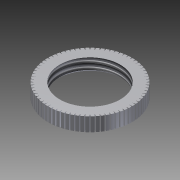
# Autodesk Inventor part: AT504M
Saved by Autodesk Inventor 2011 SP1 (Build 150282100, 282)
## iProperties
Created: 2013-12-24
Part Number: AT504M
Catalog Web Link: www.cadenas.de
Description: AT504M-Knurled Face Nut
Vendor: NKKSWITCHES
Document SubType Name: Modeling
Designer: PARTuser1
Manufacturer: NKKSWITCHES
Density: 1 g/cm^3
Category: PARTsolutions
Company: NKKSWITCHES
Title: AT504M
Author: Cadenas PARTsolutions
Comments: Knurled Face Nut
PSOL_IDENT_0: {$CADENAS_DATA\23d-libs\nkkswitches\toggle\s\parts\at504m.prj},154 {VTYP=3D},{NB=AT504M},{LINA=AT504
PSOL_IDENT_1: M},{NN=AT504M},{DATE=05.04.2013 11:05:33},{GEOMDATE=05.04.2013 12:59:00},{VERSION=},{LINEID=10},{LIN
PSOL_IDENT_2: ESUBID=-1},{WBVAR=}  {NB=AT504M},{LINA=AT504M},{KT=DUMMY},{PN=AT504M}
CNS_NN: AT504M
CNS_NT: Knurled Face Nut
CNS_NB: AT504M
CNS_NBSYN: $PN.
CNS_LINA: AT504M
CNS_PN: AT504M
SUPPLIER: NKKSWITCHES
ARTICLENO: AT504M
BOMINFO: AT504M
CREATOR: CADENAS GmbH
Autodesk Inventor part; units mm, degrees
sketch "Sketch_1" plane through (0, 0, 0) normal (0, 1, 0) x (-1, 0, 0)
  circle A0 centre (0, 0) radius 7.5946
  constraints: 1 centre point
extrude "Extrusion1" add sketch "Sketch_1" along normal blind 2.4892
sketch "Sketch2" plane through (0, 0, 0) normal (0, -1, 0) x (1, 0, 0)
  point P0 (0, 0)
hole "Drilling 1" at (0, 0, 0) direction (0, 1, 0) diameter 10.917 depth 2.4892 countersink diameter 12 countersink angle 90 thread size "M12x1" class "6H" standard "ISO Metric profile"
sketch "Sketch_3" plane through (0, 0, 0) normal (0, 1, 0) x (-1, 0, 0)
  circle A0 centre (0, 0) radius 8.89
  line L0 (8.2525, -0.2011) -> (7.112, 0)
  line L1 (7.112, 0) -> (8.2525, 0.2011)
  arc A1 (8.2525, 0.2011) -> (8.2387, 0.5189) centre (0, 0) ccw
  line L2 (8.2387, 0.5189) -> (7.0849, 0.6199)
  line L3 (7.0849, 0.6199) -> (8.2036, 0.9196)
  arc A2 (8.2036, 0.9196) -> (8.1621, 1.235) centre (0, 0) ccw
  line L4 (8.1621, 1.235) -> (7.004, 1.235)
  line L5 (7.004, 1.235) -> (8.0923, 1.6311)
  arc A3 (8.0923, 1.6311) -> (8.0234, 1.9417) centre (0, 0) ccw
  line L6 (8.0234, 1.9417) -> (6.8697, 1.8407)
  line L7 (6.8697, 1.8407) -> (7.9193, 2.3302)
  arc A4 (7.9193, 2.3302) -> (7.8236, 2.6336) centre (0, 0) ccw
  line L8 (7.8236, 2.6336) -> (6.6831, 2.4324)
  line L9 (6.6831, 2.4324) -> (7.6861, 3.0115)
  arc A5 (7.6861, 3.0115) -> (7.5643, 3.3054) centre (0, 0) ccw
  line L10 (7.5643, 3.3054) -> (6.4457, 3.0057)
  line L11 (6.4457, 3.0057) -> (7.3944, 3.6699)
  arc A6 (7.3944, 3.6699) -> (7.2475, 3.9521) centre (0, 0) ccw
  line L12 (7.2475, 3.9521) -> (6.1592, 3.556)
  line L13 (6.1592, 3.556) -> (7.0464, 4.3004)
  arc A7 (7.0464, 4.3004) -> (6.8754, 4.5687) centre (0, 0) ccw
  line L14 (6.8754, 4.5687) -> (5.8258, 4.0793)
  line L15 (5.8258, 4.0793) -> (6.6447, 4.8982)
  arc A8 (6.6447, 4.8982) -> (6.4511, 5.1506) centre (0, 0) ccw
  line L16 (6.4511, 5.1506) -> (5.4481, 4.5715)
  line L17 (5.4481, 4.5715) -> (6.1925, 5.4587)
  arc A9 (6.1925, 5.4587) -> (5.9776, 5.6932) centre (0, 0) ccw
  line L18 (5.9776, 5.6932) -> (5.0289, 5.0289)
  line L19 (5.0289, 5.0289) -> (5.6932, 5.9776)
  arc A10 (5.6932, 5.9776) -> (5.4587, 6.1925) centre (0, 0) ccw
  line L20 (5.4587, 6.1925) -> (4.5715, 5.4481)
  line L21 (4.5715, 5.4481) -> (5.1506, 6.4511)
  arc A11 (5.1506, 6.4511) -> (4.8982, 6.6447) centre (0, 0) ccw
  line L22 (4.8982, 6.6447) -> (4.0793, 5.8258)
  line L23 (4.0793, 5.8258) -> (4.5687, 6.8754)
  arc A12 (4.5687, 6.8754) -> (4.3004, 7.0464) centre (0, 0) ccw
  line L24 (4.3004, 7.0464) -> (3.556, 6.1592)
  line L25 (3.556, 6.1592) -> (3.9521, 7.2475)
  arc A13 (3.9521, 7.2475) -> (3.6699, 7.3944) centre (0, 0) ccw
  line L26 (3.6699, 7.3944) -> (3.0057, 6.4457)
  line L27 (3.0057, 6.4457) -> (3.3054, 7.5643)
  arc A14 (3.3054, 7.5643) -> (3.0115, 7.6861) centre (0, 0) ccw
  line L28 (3.0115, 7.6861) -> (2.4324, 6.6831)
  line L29 (2.4324, 6.6831) -> (2.6336, 7.8236)
  arc A15 (2.6336, 7.8236) -> (2.3302, 7.9193) centre (0, 0) ccw
  line L30 (2.3302, 7.9193) -> (1.8407, 6.8697)
  line L31 (1.8407, 6.8697) -> (1.9417, 8.0234)
  arc A16 (1.9417, 8.0234) -> (1.6311, 8.0923) centre (0, 0) ccw
  line L32 (1.6311, 8.0923) -> (1.235, 7.004)
  line L33 (1.235, 7.004) -> (1.235, 8.1621)
  arc A17 (1.235, 8.1621) -> (0.9196, 8.2036) centre (0, 0) ccw
  line L34 (0.9196, 8.2036) -> (0.6199, 7.0849)
  line L35 (0.6199, 7.0849) -> (0.5189, 8.2387)
  arc A18 (0.5189, 8.2387) -> (0.2011, 8.2525) centre (0, 0) ccw
  line L36 (0.2011, 8.2525) -> (0, 7.112)
  line L37 (0, 7.112) -> (-0.2011, 8.2525)
  arc A19 (-0.2011, 8.2525) -> (-0.5189, 8.2387) centre (0, 0) ccw
  line L38 (-0.5189, 8.2387) -> (-0.6199, 7.0849)
  line L39 (-0.6199, 7.0849) -> (-0.9196, 8.2036)
  arc A20 (-0.9196, 8.2036) -> (-1.235, 8.1621) centre (0, 0) ccw
  line L40 (-1.235, 8.1621) -> (-1.235, 7.004)
  line L41 (-1.235, 7.004) -> (-1.6311, 8.0923)
  arc A21 (-1.6311, 8.0923) -> (-1.9417, 8.0234) centre (0, 0) ccw
  line L42 (-1.9417, 8.0234) -> (-1.8407, 6.8697)
  line L43 (-1.8407, 6.8697) -> (-2.3302, 7.9193)
  arc A22 (-2.3302, 7.9193) -> (-2.6336, 7.8236) centre (0, 0) ccw
  line L44 (-2.6336, 7.8236) -> (-2.4324, 6.6831)
  line L45 (-2.4324, 6.6831) -> (-3.0115, 7.6861)
  arc A23 (-3.0115, 7.6861) -> (-3.3054, 7.5643) centre (0, 0) ccw
  line L46 (-3.3054, 7.5643) -> (-3.0057, 6.4457)
  line L47 (-3.0057, 6.4457) -> (-3.6699, 7.3944)
  arc A24 (-3.6699, 7.3944) -> (-3.9521, 7.2475) centre (0, 0) ccw
  line L48 (-3.9521, 7.2475) -> (-3.556, 6.1592)
  line L49 (-3.556, 6.1592) -> (-4.3004, 7.0464)
  arc A25 (-4.3004, 7.0464) -> (-4.5687, 6.8754) centre (0, 0) ccw
  line L50 (-4.5687, 6.8754) -> (-4.0793, 5.8258)
  line L51 (-4.0793, 5.8258) -> (-4.8982, 6.6447)
  arc A26 (-4.8982, 6.6447) -> (-5.1506, 6.4511) centre (0, 0) ccw
  line L52 (-5.1506, 6.4511) -> (-4.5715, 5.4481)
  line L53 (-4.5715, 5.4481) -> (-5.4587, 6.1925)
  arc A27 (-5.4587, 6.1925) -> (-5.6932, 5.9776) centre (0, 0) ccw
  line L54 (-5.6932, 5.9776) -> (-5.0289, 5.0289)
  line L55 (-5.0289, 5.0289) -> (-5.9776, 5.6932)
  arc A28 (-5.9776, 5.6932) -> (-6.1925, 5.4587) centre (0, 0) ccw
  line L56 (-6.1925, 5.4587) -> (-5.4481, 4.5715)
  line L57 (-5.4481, 4.5715) -> (-6.4511, 5.1506)
  arc A29 (-6.4511, 5.1506) -> (-6.6447, 4.8982) centre (0, 0) ccw
  line L58 (-6.6447, 4.8982) -> (-5.8258, 4.0793)
  line L59 (-5.8258, 4.0793) -> (-6.8754, 4.5687)
  arc A30 (-6.8754, 4.5687) -> (-7.0464, 4.3004) centre (0, 0) ccw
  line L60 (-7.0464, 4.3004) -> (-6.1592, 3.556)
  line L61 (-6.1592, 3.556) -> (-7.2475, 3.9521)
  arc A31 (-7.2475, 3.9521) -> (-7.3944, 3.6699) centre (0, 0) ccw
  line L62 (-7.3944, 3.6699) -> (-6.4457, 3.0057)
  line L63 (-6.4457, 3.0057) -> (-7.5643, 3.3054)
  arc A32 (-7.5643, 3.3054) -> (-7.6861, 3.0115) centre (0, 0) ccw
  line L64 (-7.6861, 3.0115) -> (-6.6831, 2.4324)
  line L65 (-6.6831, 2.4324) -> (-7.8236, 2.6336)
  arc A33 (-7.8236, 2.6336) -> (-7.9193, 2.3302) centre (0, 0) ccw
  line L66 (-7.9193, 2.3302) -> (-6.8697, 1.8407)
  line L67 (-6.8697, 1.8407) -> (-8.0234, 1.9417)
  arc A34 (-8.0234, 1.9417) -> (-8.0923, 1.6311) centre (0, 0) ccw
  line L68 (-8.0923, 1.6311) -> (-7.004, 1.235)
  line L69 (-7.004, 1.235) -> (-8.1621, 1.235)
  arc A35 (-8.1621, 1.235) -> (-8.2036, 0.9196) centre (0, 0) ccw
  line L70 (-8.2036, 0.9196) -> (-7.0849, 0.6199)
  line L71 (-7.0849, 0.6199) -> (-8.2387, 0.5189)
  arc A36 (-8.2387, 0.5189) -> (-8.2525, 0.2011) centre (0, 0) ccw
  line L72 (-8.2525, 0.2011) -> (-7.112, 0)
  line L73 (-7.112, 0) -> (-8.2525, -0.2011)
  arc A37 (-8.2525, -0.2011) -> (-8.2387, -0.5189) centre (0, 0) ccw
  line L74 (-8.2387, -0.5189) -> (-7.0849, -0.6199)
  line L75 (-7.0849, -0.6199) -> (-8.2036, -0.9196)
  arc A38 (-8.2036, -0.9196) -> (-8.1621, -1.235) centre (0, 0) ccw
  line L76 (-8.1621, -1.235) -> (-7.004, -1.235)
  line L77 (-7.004, -1.235) -> (-8.0923, -1.6311)
  arc A39 (-8.0923, -1.6311) -> (-8.0234, -1.9417) centre (0, 0) ccw
  line L78 (-8.0234, -1.9417) -> (-6.8697, -1.8407)
  line L79 (-6.8697, -1.8407) -> (-7.9193, -2.3302)
  arc A40 (-7.9193, -2.3302) -> (-7.8236, -2.6336) centre (0, 0) ccw
  line L80 (-7.8236, -2.6336) -> (-6.6831, -2.4324)
  line L81 (-6.6831, -2.4324) -> (-7.6861, -3.0115)
  arc A41 (-7.6861, -3.0115) -> (-7.5643, -3.3054) centre (0, 0) ccw
  line L82 (-7.5643, -3.3054) -> (-6.4457, -3.0057)
  line L83 (-6.4457, -3.0057) -> (-7.3944, -3.6699)
  arc A42 (-7.3944, -3.6699) -> (-7.2475, -3.9521) centre (0, 0) ccw
  line L84 (-7.2475, -3.9521) -> (-6.1592, -3.556)
  line L85 (-6.1592, -3.556) -> (-7.0464, -4.3004)
  arc A43 (-7.0464, -4.3004) -> (-6.8754, -4.5687) centre (0, 0) ccw
  line L86 (-6.8754, -4.5687) -> (-5.8258, -4.0793)
  line L87 (-5.8258, -4.0793) -> (-6.6447, -4.8982)
  arc A44 (-6.6447, -4.8982) -> (-6.4511, -5.1506) centre (0, 0) ccw
  line L88 (-6.4511, -5.1506) -> (-5.4481, -4.5715)
  line L89 (-5.4481, -4.5715) -> (-6.1925, -5.4587)
  arc A45 (-6.1925, -5.4587) -> (-5.9776, -5.6932) centre (0, 0) ccw
  line L90 (-5.9776, -5.6932) -> (-5.0289, -5.0289)
  line L91 (-5.0289, -5.0289) -> (-5.6932, -5.9776)
  arc A46 (-5.6932, -5.9776) -> (-5.4587, -6.1925) centre (0, 0) ccw
  line L92 (-5.4587, -6.1925) -> (-4.5715, -5.4481)
  line L93 (-4.5715, -5.4481) -> (-5.1506, -6.4511)
  arc A47 (-5.1506, -6.4511) -> (-4.8982, -6.6447) centre (0, 0) ccw
  line L94 (-4.8982, -6.6447) -> (-4.0793, -5.8258)
  line L95 (-4.0793, -5.8258) -> (-4.5687, -6.8754)
  arc A48 (-4.5687, -6.8754) -> (-4.3004, -7.0464) centre (0, 0) ccw
  line L96 (-4.3004, -7.0464) -> (-3.556, -6.1592)
  line L97 (-3.556, -6.1592) -> (-3.9521, -7.2475)
  arc A49 (-3.9521, -7.2475) -> (-3.6699, -7.3944) centre (0, 0) ccw
  line L98 (-3.6699, -7.3944) -> (-3.0057, -6.4457)
  line L99 (-3.0057, -6.4457) -> (-3.3054, -7.5643)
  arc A50 (-3.3054, -7.5643) -> (-3.0115, -7.6861) centre (0, 0) ccw
  line L100 (-3.0115, -7.6861) -> (-2.4324, -6.6831)
  line L101 (-2.4324, -6.6831) -> (-2.6336, -7.8236)
  arc A51 (-2.6336, -7.8236) -> (-2.3302, -7.9193) centre (0, 0) ccw
  line L102 (-2.3302, -7.9193) -> (-1.8407, -6.8697)
  line L103 (-1.8407, -6.8697) -> (-1.9417, -8.0234)
  arc A52 (-1.9417, -8.0234) -> (-1.6311, -8.0923) centre (0, 0) ccw
  line L104 (-1.6311, -8.0923) -> (-1.235, -7.004)
  line L105 (-1.235, -7.004) -> (-1.235, -8.1621)
  arc A53 (-1.235, -8.1621) -> (-0.9196, -8.2036) centre (0, 0) ccw
  line L106 (-0.9196, -8.2036) -> (-0.6199, -7.0849)
  line L107 (-0.6199, -7.0849) -> (-0.5189, -8.2387)
  arc A54 (-0.5189, -8.2387) -> (-0.2011, -8.2525) centre (0, 0) ccw
  line L108 (-0.2011, -8.2525) -> (0, -7.112)
  line L109 (0, -7.112) -> (0.2011, -8.2525)
  arc A55 (0.2011, -8.2525) -> (0.5189, -8.2387) centre (0, 0) ccw
  line L110 (0.5189, -8.2387) -> (0.6199, -7.0849)
  line L111 (0.6199, -7.0849) -> (0.9196, -8.2036)
  arc A56 (0.9196, -8.2036) -> (1.235, -8.1621) centre (0, 0) ccw
  line L112 (1.235, -8.1621) -> (1.235, -7.004)
  line L113 (1.235, -7.004) -> (1.6311, -8.0923)
  arc A57 (1.6311, -8.0923) -> (1.9417, -8.0234) centre (0, 0) ccw
  line L114 (1.9417, -8.0234) -> (1.8407, -6.8697)
  line L115 (1.8407, -6.8697) -> (2.3302, -7.9193)
  arc A58 (2.3302, -7.9193) -> (2.6336, -7.8236) centre (0, 0) ccw
  line L116 (2.6336, -7.8236) -> (2.4324, -6.6831)
  line L117 (2.4324, -6.6831) -> (3.0115, -7.6861)
  arc A59 (3.0115, -7.6861) -> (3.3054, -7.5643) centre (0, 0) ccw
  line L118 (3.3054, -7.5643) -> (3.0057, -6.4457)
  line L119 (3.0057, -6.4457) -> (3.6699, -7.3944)
  arc A60 (3.6699, -7.3944) -> (3.9521, -7.2475) centre (0, 0) ccw
  line L120 (3.9521, -7.2475) -> (3.556, -6.1592)
  line L121 (3.556, -6.1592) -> (4.3004, -7.0464)
  arc A61 (4.3004, -7.0464) -> (4.5687, -6.8754) centre (0, 0) ccw
  line L122 (4.5687, -6.8754) -> (4.0793, -5.8258)
  line L123 (4.0793, -5.8258) -> (4.8982, -6.6447)
  arc A62 (4.8982, -6.6447) -> (5.1506, -6.4511) centre (0, 0) ccw
  line L124 (5.1506, -6.4511) -> (4.5715, -5.4481)
  line L125 (4.5715, -5.4481) -> (5.4587, -6.1925)
  arc A63 (5.4587, -6.1925) -> (5.6932, -5.9776) centre (0, 0) ccw
  line L126 (5.6932, -5.9776) -> (5.0289, -5.0289)
  line L127 (5.0289, -5.0289) -> (5.9776, -5.6932)
  arc A64 (5.9776, -5.6932) -> (6.1925, -5.4587) centre (0, 0) ccw
  line L128 (6.1925, -5.4587) -> (5.4481, -4.5715)
  line L129 (5.4481, -4.5715) -> (6.4511, -5.1506)
  arc A65 (6.4511, -5.1506) -> (6.6447, -4.8982) centre (0, 0) ccw
  line L130 (6.6447, -4.8982) -> (5.8258, -4.0793)
  line L131 (5.8258, -4.0793) -> (6.8754, -4.5687)
  arc A66 (6.8754, -4.5687) -> (7.0464, -4.3004) centre (0, 0) ccw
  line L132 (7.0464, -4.3004) -> (6.1592, -3.556)
  line L133 (6.1592, -3.556) -> (7.2475, -3.9521)
  arc A67 (7.2475, -3.9521) -> (7.3944, -3.6699) centre (0, 0) ccw
  line L134 (7.3944, -3.6699) -> (6.4457, -3.0057)
  line L135 (6.4457, -3.0057) -> (7.5643, -3.3054)
  arc A68 (7.5643, -3.3054) -> (7.6861, -3.0115) centre (0, 0) ccw
  line L136 (7.6861, -3.0115) -> (6.6831, -2.4324)
  line L137 (6.6831, -2.4324) -> (7.8236, -2.6336)
  arc A69 (7.8236, -2.6336) -> (7.9193, -2.3302) centre (0, 0) ccw
  line L138 (7.9193, -2.3302) -> (6.8697, -1.8407)
  line L139 (6.8697, -1.8407) -> (8.0234, -1.9417)
  arc A70 (8.0234, -1.9417) -> (8.0923, -1.6311) centre (0, 0) ccw
  line L140 (8.0923, -1.6311) -> (7.004, -1.235)
  line L141 (7.004, -1.235) -> (8.1621, -1.235)
  arc A71 (8.1621, -1.235) -> (8.2036, -0.9196) centre (0, 0) ccw
  line L142 (8.2036, -0.9196) -> (7.0849, -0.6199)
  line L143 (7.0849, -0.6199) -> (8.2387, -0.5189)
  arc A72 (8.2387, -0.5189) -> (8.2525, -0.2011) centre (0, 0) ccw
  constraints: 288 end point, 144 point on circle, 73 centre point
extrude "Extrusion2" cut sketch "Sketch_3" along normal blind 2.4892
ref_plane "b_XY" through (0, 0, 0) normal (0, -1, 0) x (1, 0, 0)
ref_plane "b_YZ" through (0, 0, 0) normal (1, 0, 0) x (0, 0, 1)
ref_plane "b_ZX" through (0, 0, 0) normal (0, 0, 1) x (0, -1, 0)
ref_plane "t_XY" through (0, 2.4892, 0) normal (0, 1, 0) x (1, 0, 0)
ref_plane "t_YZ" through (0, 2.4892, 0) normal (1, 0, 0) x (0, 0, -1)
ref_plane "t_ZX" through (0, 2.4892, 0) normal (0, 0, -1) x (0, 1, 0)
body "Solid1"
